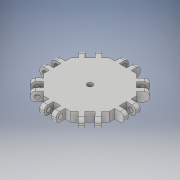
# Autodesk Inventor part: Hex_Center
Saved by Autodesk Inventor 2019 (Build 230136000, 136)
## iProperties
Created: 2019-11-16
Part Number: Hex_Center
Material: Generic
Document SubType Name: Modeling
Designer: Jorian Brusind
Density: 1 g/cm^3
Appearance: Default
Author: Jorian Brusind
Autodesk Inventor part; units mm, degrees
ref_plane "YZ Plane" through (0, 0, 0) normal (1, 0, 0) x (0, 1, 0)
ref_plane "XZ Plane" through (0, 0, 0) normal (0, 1, 0) x (-1, 0, 0)
ref_plane "XY Plane" through (0, 0, 0) normal (0, 0, 1) x (1, 0, 0)
sketch "Sketch1" plane through (0, 0, 0) normal (0, 1, 0) x (-1, 0, 0)
  line L0 (18.1266, 7.4516) -> (18.0866, -7.5484)
  line L1 (18.0866, -7.5484) -> (7.4516, -18.1266)
  line L2 (7.4516, -18.1266) -> (-7.5484, -18.0866)
  line L3 (-7.5484, -18.0866) -> (-18.1266, -7.4516)
  line L4 (-18.1266, -7.4516) -> (-18.0866, 7.5484)
  line L5 (-18.0866, 7.5484) -> (-7.4516, 18.1266)
  line L6 (-7.4516, 18.1266) -> (7.5484, 18.0866)
  line L7 (7.5484, 18.0866) -> (18.1266, 7.4516)
  point P0 (0, 0)
  point P1 (0, 0)
  dimension "d0" = 15
  dimension "d20" = 10.5783
  constraints: 16 end point, 1 coincident, 17 other
  measures "d0" vertical distance of L0.start L0.end
  measures "d20" horizontal distance of L6.end L0.start
extrude "Extrusion1" add sketch "Sketch1" along normal blind 5
sketch "Sketch2" plane through (0, 5, 0) normal (0, 1, 0) x (1, 0, 0)
  circle A0 centre (0, 0) radius 1.5
  dimension "d4" = 3
  constraints: 1 centre point, 1 coincident
  measures "d4" diameter of A0
extrude "Extrusion2" cut sketch "Sketch2" against normal blind 5
sketch "Sketch3" plane through (18.0866, 0, 7.5484) normal (0.7052142, 0, 0.7089943) x (0.7089943, 0, -0.7052142)
  line L0 (-15.0001, 5) -> (-12.0001, 5)
  line L1 (0, 5) -> (-15.0001, 5) projected
  line L2 (0, 5) -> (-3, 5)
  line L3 (-12.0001, 5) -> (-9.5001, 5)
  line L4 (-9.5001, 5) -> (-9.5001, 0)
  line L5 (-9.5001, 0) -> (-12.0001, 0)
  line L6 (-12.0001, 0) -> (-12.0001, 5)
  line L7 (-15.0001, 0) -> (0, 0) projected
  line L8 (-3, 5) -> (-5.5, 5)
  line L9 (-5.5, 5) -> (-5.5, 0)
  line L10 (-5.5, 0) -> (-3, 0)
  line L11 (-3, 0) -> (-3, 5)
  dimension "d21" = 3
  dimension "d22" = 3
  dimension "d23" = 2.5
  dimension "d24" = 5
  dimension "d25" = 2.5
  constraints: 20 end point, 4 parallel, 3 point on line, 2 horizontal, 2 perpendicular
  measures "d21" distance of L0.start L0.end
  measures "d22" distance of L1.start L2.end
  measures "d23" distance of L4.end L5.end
  measures "d24" distance of L3.end L4.end
  measures "d25" distance of L10.end L9.end
extrude "Extrusion5" add sketch "Sketch3" along normal blind 5 contours L11 L7 L9 L1 | L4 L5 L6 L1
sketch "Sketch5" plane through (15.9596, 0, 9.664) normal (0.7089943, 0, -0.7052142) x (-0.7052142, 0, -0.7089943)
  line L0 (0, 0) -> (-5, 0) projected
  line L1 (-5, 0) -> (-2.5, 0)
  line L2 (-2.5, 0) -> (-2.5, 2.5)
  circle A0 centre (-2.5, 2.5) radius 1.25
  point P0 (18.1067, 0)
  dimension "d28" = 2.5
  dimension "d29" = 2.5
  constraints: 4 end point, 1 centre point, 1 coincident, 1 midpoint, 1 vertical
  measures "d28" distance of L1.end L2.end
  measures "d29" diameter of A0
extrude "Extrusion6" cut sketch "Sketch5" against normal blind 8
fillet "Fillet1" radius 2 4 edges at (18.5994, 5, 14.0905) (18.5994, 0, 14.0905) (13.9909, 0, 18.6745) (13.9909, 5, 18.6745)
pattern_circular "Circular Pattern2" count 8 over 360 about axis through (0, 5, 0) along (0, -1, 0) of "Extrusion6", "Extrusion5", "Fillet1"
body "Solid1"
